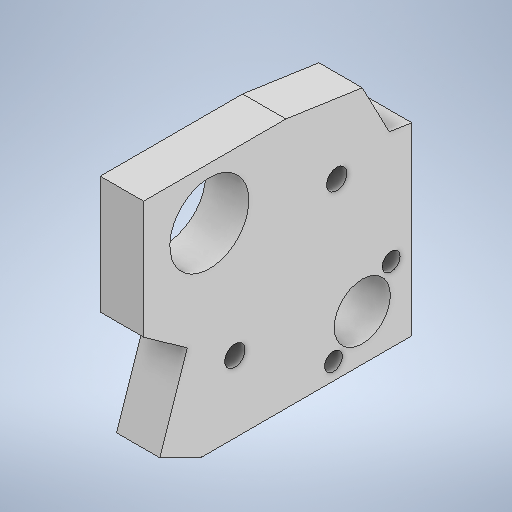
# Autodesk Inventor part: GuideBlock
Saved by Autodesk Inventor 2025.3 (Build 293356030, 356C)
## iProperties
Created: 2025-09-01
Part Number: GuideBlock
Material: Generic
Document SubType Name: Modeling
Designer: tvoko
Density: 1 g/cm^3
Appearance: Default
Author: tvoko
Autodesk Inventor part; units mm, degrees
ref_plane "YZ Plane" through (0, 0, 0) normal (1, 0, 0) x (0, 1, 0)
ref_plane "XZ Plane" through (0, 0, 0) normal (0, 1, 0) x (-1, 0, 0)
ref_plane "XY Plane" through (0, 0, 0) normal (0, 0, 1) x (1, 0, 0)
sketch "Sketch1" plane through (0, 0, 0) normal (1, 0, 0) x (0, 1, 0)
  circle A0 centre (10, -10) radius 2
  circle A1 centre (-10, 10) radius 2
  circle A2 centre (15, 15) radius 7.75
  circle A3 centre (-15, -15) radius 5.5
  line L0 (-9.3431, -20.6569) -> (-20.6569, -9.3431) construction
  circle A4 centre (10, -10) radius 6.5
  circle A5 centre (-10, 10) radius 6.5
  circle A6 centre (-9.3431, -20.6569) radius 1.75
  circle A7 centre (-20.6569, -9.3431) radius 1.75
  line L1 (-10, 10) -> (10, -10) construction
  line L2 (15, 15) -> (-15, -15) construction
  line L3 (12.214, -24.7059) -> (-23.9902, -24.7059)
  line L4 (-23.9902, -24.7059) -> (-23.9902, 16.5)
  line L5 (2.099, 27.901) -> (25.1854, 27.901)
  line L6 (25.1854, 27.901) -> (25.1854, -0.0328)
  line L7 (2.099, 27.901) -> (-4.0315, 19.3184)
  line L8 (-4.0315, 19.3184) -> (-20, 24.7124)
  line L9 (-20, 24.7124) -> (-23.9902, 16.5)
  line L10 (12.214, -24.7059) -> (12.8582, -20.2942)
  line L11 (12.8582, -20.2942) -> (23, -15)
  line L12 (23, -15) -> (25.1854, -0.0328)
  point P0 (0, 0)
  point P1 (0, 0)
  dimension "d0" = 4
  dimension "d2" = 13
  dimension "d3" = 16
  dimension "d4" = 11
  dimension "d5" = 3.5
  dimension "d6" = 20
  dimension "d7" = 20
  dimension "d8" = 30
  dimension "d9" = 30
  dimension "d10" = 15.5
  constraints: 27 end point, 8 centre point, 6 coincident, 4 perpendicular, 3 equal radius, 3 midpoint, 1 horizontal, 1 parallel
  measures "d0" diameter of A0
  measures "d2" diameter of A4
  measures "d3" distance of L0.start L0.end
  measures "d4" diameter of A3
  measures "d5" diameter of A6
  measures "d6" horizontal distance of A1.centre A0.centre
  measures "d7" horizontal distance of A1.centre A0.centre
  measures "d8" horizontal distance of A3.centre L2.start
  measures "d9" horizontal distance of L2.start A3.centre
  measures "d10" diameter of A2
extrude "Extrusion1" add sketch "Sketch1" against normal blind 8.5 contours A4 | A5 | L3 L4 L9 L8 L7 L5 L6 L12 L11 L10
body "Solid1"
